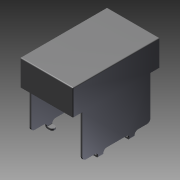
# Autodesk Inventor part: MB2011c
Saved by Autodesk Inventor 2015 (Build 190159000, 159)
## iProperties
Category: PARTsolutions
Company: NKKSWITCHES
Created: 2015-01-04
Part Number: MB2011c
Catalog Web Link: www.cadenas.de
Description: MB2000 Series - Bushing Mount Miniature Pushbuttons -body_cover-
Vendor: NKKSWITCHES
Document SubType Name: Modeling
Designer: PARTuser1
Manufacturer: NKKSWITCHES
Mass: 0.0970001 g
Surface Area: 7.81178 cm^2
Volume: 0.0970001 cm^3
Density: 1 g/cm^3
Material: Generic
Appearance: PSOLRGB-242-242-242
PSOL_IDENT_0: {$CADENAS_DATA\23d-libs\nkkswitches\pushbuttons\mb2000\parts\mb2000_body_cover.prj},221 {VTYP=3D},{N
PSOL_IDENT_1: B=MB2011c},{LINA=MB2011c},{NN=MB2000 Series - Bushing Mount Miniature Pushbuttons -body_cover},{DATE=
PSOL_IDENT_2: 21.11.2014 08:56:24},{GEOMDATE=12.01.2009 00:00:00},{VERSION=},{LINEID=10},{LINESUBID=-1},{WBVAR=PLS
PSOL_IDENT_3: CRCTS}  {NB=MB2011c},{LINA=MB2011c},{KT=DUMMY},{PN=MB2011},{SRS=MB},{PLSCRCTS=2011}
SUPPLIER: NKKSWITCHES
ARTICLENO: MB2011c
BOMINFO: MB2011c
CREATOR: CADENAS GmbH
Title: MB2011c
Author: Cadenas PARTsolutions
Autodesk Inventor part; units mm, degrees
sketch "Sketch_1" plane through (0, 0, 0) normal (0, 1, 0) x (-1, 0, 0)
  line L0 (3.9497, -6.3754) -> (3.9497, 6.3754)
  arc A0 (3.9497, 6.3754) -> (3.8227, 6.5024) centre (3.8227, 6.3754) ccw
  line L1 (3.8227, 6.5024) -> (-3.8227, 6.5024)
  arc A1 (-3.8227, 6.5024) -> (-3.9497, 6.3754) centre (-3.8227, 6.3754) ccw
  line L2 (-3.9497, 6.3754) -> (-3.9497, -6.3754)
  arc A2 (-3.9497, -6.3754) -> (-3.8227, -6.5024) centre (-3.8227, -6.3754) ccw
  line L3 (-3.8227, -6.5024) -> (3.8227, -6.5024)
  arc A3 (3.8227, -6.5024) -> (3.9497, -6.3754) centre (3.8227, -6.3754) ccw
  line L4 (3.6957, -6.2484) -> (3.6957, 6.2484)
  line L5 (3.6957, 6.2484) -> (-3.6957, 6.2484)
  line L6 (-3.6957, 6.2484) -> (-3.6957, -6.2484)
  line L7 (-3.6957, -6.2484) -> (3.6957, -6.2484)
  constraints: 16 end point, 8 point on circle, 4 centre point
extrude "Extrusion1" add sketch "Sketch_1" against normal blind 3.5814
sketch "Sketch_2" plane through (0, 0, 0) normal (0, 1, 0) x (-1, 0, 0)
  line L0 (3.9497, -6.3754) -> (3.9497, 6.3754)
  arc A0 (3.9497, 6.3754) -> (3.8227, 6.5024) centre (3.8227, 6.3754) ccw
  line L1 (3.8227, 6.5024) -> (-3.8227, 6.5024)
  arc A1 (-3.8227, 6.5024) -> (-3.9497, 6.3754) centre (-3.8227, 6.3754) ccw
  line L2 (-3.9497, 6.3754) -> (-3.9497, -6.3754)
  arc A2 (-3.9497, -6.3754) -> (-3.8227, -6.5024) centre (-3.8227, -6.3754) ccw
  line L3 (-3.8227, -6.5024) -> (3.8227, -6.5024)
  arc A3 (3.8227, -6.5024) -> (3.9497, -6.3754) centre (3.8227, -6.3754) ccw
  constraints: 8 end point, 8 point on circle, 4 centre point
extrude "Extrusion2" add sketch "Sketch_2" along normal blind 0.254
sketch "Sketch_7" plane through (0, 0, 0) normal (0, 0, 1) x (1, 0, 0)
  line L0 (-3.9497, 0.4023) -> (-3.9497, 0.127)
  arc A0 (-3.8227, 0.254) -> (-3.9497, 0.127) centre (-3.8227, 0.127) ccw
  line L1 (-3.8227, 0.254) -> (3.8227, 0.254)
  arc A1 (3.9497, 0.127) -> (3.8227, 0.254) centre (3.8227, 0.127) ccw
  line L2 (3.9497, 0.127) -> (3.9497, 0.4023)
  line L3 (3.9497, 0.4023) -> (-3.9497, 0.4023)
  constraints: 8 end point, 4 point on circle, 2 centre point
extrude "Extrusion3" cut sketch "Sketch_7" along normal mid plane 15.24
sketch "Sketch_8" plane through (0, 0, 0) normal (1, 0, 0) x (0, 1, 0)
  line L0 (0.4023, 6.5024) -> (0.127, 6.5024)
  arc A0 (0.254, 6.3754) -> (0.127, 6.5024) centre (0.127, 6.3754) ccw
  line L1 (0.254, 6.3754) -> (0.254, -6.3754)
  arc A1 (0.127, -6.5024) -> (0.254, -6.3754) centre (0.127, -6.3754) ccw
  line L2 (0.127, -6.5024) -> (0.4023, -6.5024)
  line L3 (0.4023, -6.5024) -> (0.4023, 6.5024)
  constraints: 8 end point, 4 point on circle, 2 centre point
extrude "Extrusion4" cut sketch "Sketch_8" along normal mid plane 15.24
sketch "Sketch_13" plane through (0, 0, 0) normal (1, 0, 0) x (0, 1, 0)
  line L0 (-3.5814, 5.08) -> (-9.4403, 5.08)
  arc A0 (-9.4403, 5.08) -> (-9.9483, 4.572) centre (-9.4403, 4.572) ccw
  line L1 (-9.9483, 4.572) -> (-9.9483, 3.2258)
  arc A1 (-10.4563, 2.7178) -> (-9.9483, 3.2258) centre (-10.4563, 3.2258) ccw
  line L2 (-10.4563, 2.7178) -> (-10.7103, 2.7178)
  line L3 (-10.7103, 2.7178) -> (-10.7103, 1.9558)
  line L4 (-10.7103, 1.9558) -> (-10.4563, 1.9558)
  arc A2 (-9.9483, 1.4478) -> (-10.4563, 1.9558) centre (-10.4563, 1.4478) ccw
  line L5 (-9.9483, 1.4478) -> (-9.9483, -1.4478)
  arc A3 (-10.4563, -1.9558) -> (-9.9483, -1.4478) centre (-10.4563, -1.4478) ccw
  line L6 (-10.4563, -1.9558) -> (-10.7103, -1.9558)
  line L7 (-10.7103, -1.9558) -> (-10.7103, -2.7178)
  line L8 (-10.7103, -2.7178) -> (-10.4563, -2.7178)
  arc A4 (-9.9483, -3.2258) -> (-10.4563, -2.7178) centre (-10.4563, -3.2258) ccw
  line L9 (-9.9483, -3.2258) -> (-9.9483, -4.572)
  arc A5 (-9.9483, -4.572) -> (-9.4403, -5.08) centre (-9.4403, -4.572) ccw
  line L10 (-9.4403, -5.08) -> (-3.5814, -5.08)
  line L11 (-3.5814, -5.08) -> (-3.5814, 5.08)
  constraints: 24 end point, 12 point on circle, 6 centre point
extrude "Extrusion5" add sketch "Sketch_13" along normal mid plane 7.8994
sketch "Sketch_14" plane through (0, 0, 0) normal (0, 0, 1) x (1, 0, 0)
  line L0 (-3.9497, -11.1282) -> (3.9497, -11.1282)
  line L1 (3.9497, -11.1282) -> (3.9497, -10.4563)
  arc A0 (3.6957, -10.7103) -> (3.9497, -10.4563) centre (3.6957, -10.4563) ccw
  line L2 (3.6957, -10.7103) -> (3.3147, -10.7103)
  line L3 (3.3147, -10.7103) -> (3.3147, -10.4563)
  line L4 (3.3147, -10.4563) -> (3.6322, -10.4563)
  arc A1 (3.6322, -10.4563) -> (3.6957, -10.3928) centre (3.6322, -10.3928) ccw
  line L5 (3.6957, -10.3928) -> (3.6957, -3.5814)
  line L6 (3.6957, -3.5814) -> (-3.6957, -3.5814)
  line L7 (-3.6957, -3.5814) -> (-3.6957, -10.3928)
  arc A2 (-3.6957, -10.3928) -> (-3.6322, -10.4563) centre (-3.6322, -10.3928) ccw
  line L8 (-3.6322, -10.4563) -> (-3.3147, -10.4563)
  line L9 (-3.3147, -10.4563) -> (-3.3147, -10.7103)
  line L10 (-3.3147, -10.7103) -> (-3.6957, -10.7103)
  arc A3 (-3.9497, -10.4563) -> (-3.6957, -10.7103) centre (-3.6957, -10.4563) ccw
  line L11 (-3.9497, -10.4563) -> (-3.9497, -11.1282)
  constraints: 24 end point, 8 point on circle, 4 centre point
extrude "Extrusion6" cut sketch "Sketch_14" along normal mid plane 10.287
sketch "Sketch_29" plane through (-3.6957, -10.7103, 1.9558) normal (0, -1, 0) x (1, 0, 0)
  line L0 (0, 0.762) -> (0, 0)
  line L1 (0, 0) -> (0.381, 0)
  arc A0 (0.381, 0) -> (0.381, 0.762) centre (0.381, 0.381) ccw
  line L2 (0.381, 0.762) -> (0, 0.762)
  constraints: 6 end point, 2 point on circle, 1 centre point
extrude "Extrusion7" add sketch "Sketch_29" against normal blind 0.254
sketch "Sketch_30" plane through (-3.6957, -10.7103, 1.9558) normal (0, -1, 0) x (1, 0, 0)
  arc A0 (7.0104, 0.762) -> (7.0104, 0) centre (7.0104, 0.381) ccw
  line L0 (7.0104, 0) -> (7.3914, 0)
  line L1 (7.3914, 0) -> (7.3914, 0.762)
  line L2 (7.3914, 0.762) -> (7.0104, 0.762)
  constraints: 6 end point, 2 point on circle, 1 centre point
extrude "Extrusion8" add sketch "Sketch_30" against normal blind 0.254
sketch "Sketch_31" plane through (-3.6957, -10.7103, -2.7178) normal (0, -1, 0) x (1, 0, 0)
  line L0 (0, 0.762) -> (0, 0)
  line L1 (0, 0) -> (0.381, 0)
  arc A0 (0.381, 0) -> (0.381, 0.762) centre (0.381, 0.381) ccw
  line L2 (0.381, 0.762) -> (0, 0.762)
  constraints: 6 end point, 2 point on circle, 1 centre point
extrude "Extrusion9" add sketch "Sketch_31" against normal blind 0.254
sketch "Sketch_32" plane through (-3.6957, -10.7103, -2.7178) normal (0, -1, 0) x (1, 0, 0)
  arc A0 (7.0104, 0.762) -> (7.0104, 0) centre (7.0104, 0.381) ccw
  line L0 (7.0104, 0) -> (7.3914, 0)
  line L1 (7.3914, 0) -> (7.3914, 0.762)
  line L2 (7.3914, 0.762) -> (7.0104, 0.762)
  constraints: 6 end point, 2 point on circle, 1 centre point
extrude "Extrusion10" add sketch "Sketch_32" against normal blind 0.254
ref_plane "to_body_XY" through (0, 0, 0) normal (0, 1, 0) x (1, 0, 0)
ref_plane "to_body_YZ" through (0, 0, 0) normal (1, 0, 0) x (0, 0, -1)
ref_plane "to_body_ZX" through (0, 0, 0) normal (0, 0, -1) x (0, 1, 0)
ref_plane "to_bushings_XY" through (0, 0.254, 0) normal (0, -1, 0) x (1, 0, 0)
ref_plane "to_bushings_YZ" through (0, 0.254, 0) normal (1, 0, 0) x (0, 0, 1)
ref_plane "to_bushings_ZX" through (0, 0.254, 0) normal (0, 0, 1) x (0, -1, 0)
body "Solid1"
